Autodesk Fusion 360 part; units mm, degrees
(part 2 of 2)
sketch "Esquisse3" plane through (0, 0, -1.5) normal (0, 0, -1) x (1, 0, 0)
  line L0 (-2, 0) -> (11.5, 0)
  line L1 (11.5, 0) -> (11.5, 12)
  line L2 (11.5, 12) -> (-2, 12)
  line L3 (-2, 12) -> (-2, 0)
  line L4 (11.5, 0) -> (-2, 12) construction
  line L5 (-2, 0) -> (11.5, 12) construction
  line L6 (4.8934, 8.8362) -> (9.5227, 8.8362)
  arc A0 (4.8934, 8.8362) -> (1.989, 6.7416) centre (4.8934, 5.7754) ccw
  arc A1 (9.5227, 8.8362) -> (0.352, 9.4875) centre (4.7155, 6.037) ccw
  arc A2 (1.989, 6.7416) -> (0.352, 9.4875) centre (-200.2462, -111.9608) ccw
  arc A3 (4.736, 0.4742) -> (9.8854, 8.0906) centre (4.7155, 6.037) ccw
  line L7 (7.0507, 4.4833) -> (4.736, 0.4742)
  arc A4 (7.0507, 4.4833) -> (6.6889, 8.0459) centre (4.3999, 6.0137) ccw
  arc A5 (6.6889, 8.0459) -> (9.8854, 8.0906) centre (5.0072, 242.5379) ccw
  circle A6 centre (4.75, 6) radius 2
  dimension "d11" = 4
  constraint coincident L0.end L1.start
  constraint coincident L2.end L3.start
  constraint coincident L0.start L3.end
  constraint coincident L1.end L2.start
  constraint horizontal L6
  constraint tangent L6 A0
  constraint tangent L7 A4
  constraint midpoint L4 A6.centre
  measures "d11" diameter of A6
extrude "Extrusion3" add sketch "Esquisse3" along normal blind 1 separate body contours L6 A0 A1 A2 | A3 L7 A4 A5 | A6 makes body 2 at (8.8324, -7.0265, -1.5) makes body 3 at (1.8, -9.1077, -1.5) makes body 4 at (6.7475, -5.9003, -2.1667)
copy_body "Copier/Coller des corps1" bodies 2 makes body 5
move_body "Déplacer1" bodies 5 to x (-0.517021, 0.855973, 0) y (-0.855973, -0.517021, 0) z (0, 0, 1) at (2.0133, -13.03, 0)
